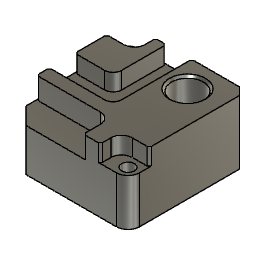
PROVA PRATICA v2 (Autodesk Fusion 360 archive; units mm, degrees)
design "PROVA PRATICA" references "okuma mb-56va"
Autodesk Fusion 360 part; units mm, degrees
sketch "Schizzo1" plane through (0, 0, 0) normal (0, 0, 1) x (1, 0, 0)
  line L0 (30, -30) -> (-30, -30)
  line L1 (-30, -30) -> (-30, 30)
  line L2 (-30, 30) -> (30, 30)
  line L3 (30, 30) -> (30, -30)
  line L4 (30, -30) -> (-30, 30) construction
  line L5 (-30, -30) -> (30, 30) construction
  line L6 (22.5, -28) -> (-22.5, -28)
  line L7 (-28, -22.5) -> (-28, 22.5)
  line L8 (-22.5, 28) -> (22.5, 28)
  line L9 (28, 22.5) -> (28, -22.5)
  arc A0 (-22.5, 28) -> (-28, 22.5) centre (-22.5, 22.5) ccw
  arc A1 (28, 22.5) -> (22.5, 28) centre (22.5, 22.5) ccw
  arc A2 (22.5, -28) -> (28, -22.5) centre (22.5, -22.5) ccw
  arc A3 (-28, -22.5) -> (-22.5, -28) centre (-22.5, -22.5) ccw
  dimension "d1" = 60
  dimension "d2" = 60
  dimension "d4" = 5.5
  constraint horizontal L0
  constraint perpendicular L0 L1
  constraint parallel L0 L2
  constraint parallel L1 L3
  constraint coincident L4 origin
  constraint coincident L5 origin
  constraint tangent L7 A0
  constraint tangent L8 A0
  constraint tangent L8 A1
  constraint tangent L9 A1
  constraint equal A0 A1
  constraint tangent L6 A2
  constraint tangent L9 A2
  constraint equal A0 A2
  constraint tangent L6 A3
  constraint tangent L7 A3
  constraint equal A0 A3
  measures "d1" distance of L1.end L2.end
  measures "d2" distance of L0.end L1.end
  measures "d4" radius of A0
extrude "Estrusione1" add sketch "Schizzo1" along normal blind 30 contours L6 L7 L8 L9 A0 A1 A2 A3
sketch "Schizzo2" plane through (0, 0, 30) normal (0, 0, 1) x (-1, 0, 0)
  arc A0 (22.5, -28) -> (28, -22.5) centre (22.5, -22.5) ccw
  line L0 (28, -22.5) -> (28, 22.5)
  arc A1 (28, 22.5) -> (22.5, 28) centre (22.5, 22.5) ccw
  line L1 (22.5, 28) -> (-22.5, 28)
  arc A2 (-22.5, 28) -> (-28, 22.5) centre (-22.5, 22.5) ccw
  line L2 (-28, 22.5) -> (-28, -22.5)
  arc A3 (-28, -22.5) -> (-22.5, -28) centre (-22.5, -22.5) ccw
  line L3 (-22.5, -28) -> (22.5, -28)
  line L4 (15, -28) -> (15, -23)
  line L5 (20, -18) -> (28, -18)
  arc A4 (20, -18) -> (15, -23) centre (20, -23) ccw
  dimension "d7" = 5
  dimension "d8" = 13
  dimension "d9" = 10
  constraint coincident L3 L4.start
  constraint perpendicular L3 L4
  constraint coincident L0 L5.end
  constraint perpendicular L0 L5
  constraint tangent L4 A4
  constraint tangent L5 A4
  measures "d7" radius of A4
  measures "d8" distance of L0 L4
  measures "d9" distance of L3 L5
extrude "Estrusione2" cut sketch "Schizzo2" against normal blind 8 contours A0 L0 L3 L4 L5 A4
pattern_circular "Serie C1" count 2 over 360 about axis through (0, 0, 1.75) along (0, 0, 1) of "Estrusione2"
sketch "Schizzo3" plane through (0, 0, 30) normal (0, 0, 1) x (-1, 0, 0)
  line L0 (-20, 18) -> (-28, 18)
  line L1 (-28, 18) -> (-28, -22.5)
  arc A0 (-28, -22.5) -> (-22.5, -28) centre (-22.5, -22.5) ccw
  line L2 (-22.5, -28) -> (15, -28)
  line L3 (15, -28) -> (15, -23)
  arc A1 (20, -18) -> (15, -23) centre (20, -23) ccw
  line L4 (20, -18) -> (28, -18)
  line L5 (28, -18) -> (28, 22.5)
  arc A2 (28, 22.5) -> (22.5, 28) centre (22.5, 22.5) ccw
  line L6 (22.5, 28) -> (-15, 28)
  line L7 (-15, 28) -> (-15, 23)
  arc A3 (-20, 18) -> (-15, 23) centre (-20, 23) ccw
  line L8 (10, -28) -> (10, -7)
  line L9 (14, -3) -> (28, -3)
  line L10 (-2, -28) -> (-2, 5)
  line L11 (2, 9) -> (28, 9)
  arc A4 (14, -3) -> (10, -7) centre (14, -7) ccw
  arc A5 (2, 9) -> (-2, 5) centre (2, 5) ccw
  circle A6 centre (-13, -15) radius 7.5
  circle A7 centre (23, -23) radius 3
  circle A8 centre (-23, 23) radius 3
  line L12 (28, 15) -> (-2, 15)
  line L13 (-7, 20) -> (-7, 28)
  arc A9 (-7, 20) -> (-2, 15) centre (-2, 20) ccw
  point P0 (-28, 18)
  dimension "d14" = 12
  dimension "d15" = 18
  dimension "d16" = 25
  dimension "d17" = 12
  dimension "d18" = 4
  dimension "d19" = 15
  dimension "d20" = 6
  dimension "d21" = 6
  dimension "d22" = 5
  dimension "d23" = 5
  dimension "d24" = 5
  dimension "d25" = 5
  dimension "d26" = 13
  dimension "d27" = 15
  dimension "d28" = 13
  dimension "d29" = 35
  dimension "d30" = 5
  constraint coincident L2 L8.start
  constraint perpendicular L2 L8
  constraint coincident L5 L9.end
  constraint perpendicular L5 L9
  constraint coincident L2 L10.start
  constraint perpendicular L2 L10
  constraint coincident L5 L11.end
  constraint perpendicular L5 L11
  constraint tangent L8 A4
  constraint tangent L9 A4
  constraint tangent L10 A5
  constraint tangent L11 A5
  constraint equal A4 A5
  constraint coincident L5 L12.start
  constraint perpendicular L5 L12
  constraint coincident L6 L13.end
  constraint perpendicular L6 L13
  constraint tangent L12 A9
  constraint tangent L13 A9
  measures "d14" distance of L8 L10
  measures "d15" distance of L5 L8
  measures "d16" distance of L2 L9
  measures "d17" distance of L9 L11
  measures "d18" radius of A4
  measures "d19" diameter of A6
  measures "d20" diameter of A7
  measures "d21" diameter of A8
  measures "d22" distance of L2 A7.centre
  measures "d23" distance of L5 A7.centre
  measures "d24" distance of L6 A8.centre
  measures "d25" horizontal distance of A8.centre P0
  measures "d26" distance of L2 A6.centre
  measures "d27" distance of L1 A6.centre
  measures "d28" distance of L6 L12
  measures "d29" distance of L5 L13
  measures "d30" radius of A9
extrude "Estrusione3" cut sketch "Schizzo3" against normal blind 85 contours A7 | A8
extrude "Estrusione4" cut sketch "Schizzo3" against normal blind 15 contours A6
extrude "Estrusione5" cut sketch "Schizzo3" against normal blind 8 contours L2 L5 L8 L9 L10 L11 A4 A5
extrude "Estrusione6" cut sketch "Schizzo3" against normal blind 10 contours L5 A2 L6 L12 L13 A9
delete_face "EliminaFaccia1" 1 faces at (-27.845, -23.7967, 13.3333)
delete_face "EliminaFaccia2" 1 faces at (26.4805, 26.2954, 20)
chamfer "Smusso1" distance 3.5 angle 45 1 edges at (28, 28, 15)
chamfer "Smusso2" distance 8 angle 45 1 edges at (-28, -28, 10)
chamfer "Smusso3" distance 1 angle 45 10 edges at (-28, -15, 25) (-28, -9, 26) (-28, 3, 26) (-28, 18, 26) (-15, 28, 26) (-10, 28, 26) (2, 28, 26) (15, -28, 26) (28, -18, 26) (7, -28, 25)
chamfer "Smusso6" distance 1 angle 45 1 edges at (19.9925, 12.2879, 30)
